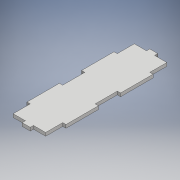
# Autodesk Inventor part: F2
Saved by Autodesk Inventor 2018 (Build 220112000, 112)
## iProperties
Created: 2018-03-06
Part Number: F2
Material: Generic
Document SubType Name: Modeling
Designer: isai
Density: 1 g/cm^3
Appearance: Default
Author: isai
Autodesk Inventor part; units mm, degrees
ref_plane "YZ Plane" through (0, 0, 0) normal (1, 0, 0) x (0, 1, 0)
ref_plane "XZ Plane" through (0, 0, 0) normal (0, 1, 0) x (-1, 0, 0)
sketch "Sketch2" plane through (0, 0, 0) normal (0, 0, 1) x (1, 0, 0)
  line L0 (29, -124.2) -> (29, -103.2)
  line L1 (29, -103.2) -> (25, -103.2)
  line L2 (25, -103.2) -> (25, -63.2)
  line L3 (25, -63.2) -> (29, -63.2)
  line L4 (29, -63.2) -> (29, -36)
  line L5 (29, -36) -> (25, -36)
  line L6 (25, -36) -> (25, 4)
  line L7 (25, 4) -> (29, 4)
  line L8 (29, 4) -> (29, 25)
  line L9 (29, 29) -> (29, 25)
  line L10 (29, 25) -> (69, 25)
  line L11 (29, -128.2) -> (29, -124.2)
  line L12 (29, -124.2) -> (69, -124.2)
  line L13 (49, -124.2) -> (49, -141.5735)
  line L14 (73, 4) -> (69, 4)
  line L15 (73, -36) -> (73, 4)
  line L16 (69, -36) -> (73, -36)
  line L17 (73, -63.2) -> (69, -63.2)
  line L18 (73, -103.2) -> (73, -63.2)
  line L19 (69, -103.2) -> (73, -103.2)
  line L20 (69, -103.2) -> (69, -124.2)
  line L21 (69, 25) -> (69, 4)
  line L22 (69, -36) -> (69, -63.2)
  point P0 (0, 0)
  dimension "d15" = 4
  dimension "d16" = 40
  dimension "d17" = 4
  dimension "d20" = 40
  dimension "d21" = 40
  dimension "d22" = 149.2
  constraints: 46 end point, 8 symmetric about line, 5 perpendicular, 1 midpoint, 1 vertical
  measures "d15" distance of L8.end L9.start
  measures "d16" distance of L8.end L10.end
  measures "d17" distance of L0.start L11.start
  measures "d20" distance of L2.start L3.start
  measures "d21" distance of L6.start L7.start
  measures "d22" distance between parallel lines of L10 L12
extrude "Extrusion3" add sketch "Sketch2" along normal blind 4
sketch "Sketch3" plane through (0, 0, 4) normal (0, 0, 1) x (1, 0, 0)
  line L0 (29, -103.2) -> (29, -124.2) projected
  line L1 (29, -124.2) -> (69, -124.2) projected
  line L2 (69, -124.2) -> (69, -103.2) projected
  line L3 (69, -103.2) -> (73, -103.2) projected
  line L4 (73, -103.2) -> (73, -63.2) projected
  line L5 (73, -63.2) -> (69, -63.2) projected
  line L6 (69, -63.2) -> (69, -36) projected
  line L7 (69, -36) -> (73, -36) projected
  line L8 (73, -36) -> (73, 4) projected
  line L9 (73, 4) -> (69, 4) projected
  line L10 (69, 4) -> (69, 25) projected
  line L11 (69, 25) -> (29, 25) projected
  line L12 (29, 25) -> (29, 4) projected
  line L13 (29, 4) -> (25, 4) projected
  line L14 (25, 4) -> (25, -36) projected
  line L15 (25, -36) -> (29, -36) projected
  line L16 (29, -36) -> (29, -63.2) projected
  line L17 (29, -63.2) -> (25, -63.2) projected
  line L18 (25, -63.2) -> (25, -103.2) projected
  line L19 (25, -103.2) -> (29, -103.2) projected
  line L20 (54, 29) -> (44, 29)
  line L21 (44, 29) -> (44, 25)
  line L22 (44, 25) -> (54, 25)
  line L23 (54, 25) -> (54, 29)
  point P0 (0, 0)
  point P1 (49, 25)
  dimension "d23" = 10
  dimension "d24" = 4
  constraints: 8 end point, 2 midpoint, 2 parallel, 1 horizontal, 1 perpendicular
  measures "d23" distance of L22.end L21.end
  measures "d24" distance of L21.end L20.end
extrude "Extrusion4" add sketch "Sketch3" against normal blind 4 contours L21 L20 L23 L11
ref_plane "Work Plane1" through (29, -49.6, 0) normal (0, -1, 0) x (1, 0, 0)
mirror "Mirror1" about plane through (29, -49.6, 0) normal (0, -1, 0) of "Extrusion4"
equation "\"d23\" = D"
equation "\"D\" = 10"
body "Solid3"
